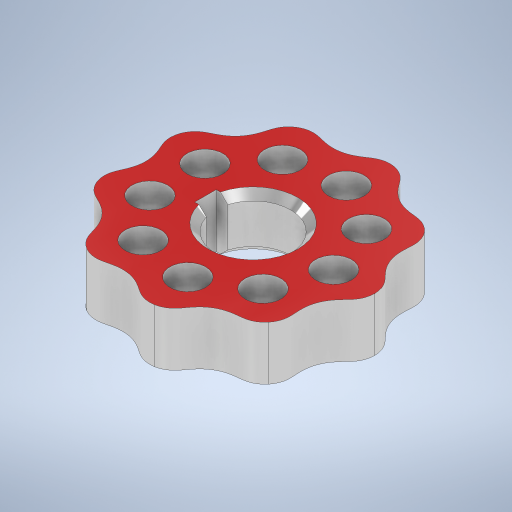
# Autodesk Inventor part: Przekładnia cykloidalna mimośrodowa
Saved by Autodesk Inventor 2023 (Build 270158000, 158)
## iProperties
Created: 2023-04-01
Part Number: Przekładnia cykloidalna mimośrodowa
Material: Stal
Document SubType Name: Modeling
Designer: Wiktor
Density: 7.85 g/cm^3
Appearance: Chrom — polerowany
Author: Wiktor
Autodesk Inventor part; units mm, degrees
ref_plane "YZ Plane" through (0, 0, 0) normal (1, 0, 0) x (0, 1, 0)
ref_plane "XZ Plane" through (0, 0, 0) normal (0, 1, 0) x (-1, 0, 0)
ref_plane "XY Plane" through (0, 0, 0) normal (0, 0, 1) x (1, 0, 0)
sketch "Szkic1" plane through (0, 0, 0) normal (0, 1, 0) x (-1, 0, 0)
  circle A0 centre (0, 0) radius 50
  dimension "d0" = 100
  constraints: 1 centre point, 1 coincident
  measures "d0" diameter of A0
extrude "Wyciągnięcie proste1" add sketch "Szkic1" along normal blind 15
sketch "Szkic2" plane through (0, 15, 0) normal (0, 1, 0) x (1, 0, 0)
  circle A0 centre (0, 0) radius 36 construction
  circle A1 centre (40, 0) radius 4 construction
  circle A2 centre (0, 0) radius 42 construction
  spline S0 degree 5 poles (42, 0) (42.0015, 1.5779) (41.7865, 3.1702) (41.3842, 4.6891) (40.322, 7.2003) (38.7977, 9.322) (38.0479, 10.2329) (36.9029, 11.2622) (35.7039, 12.7118) (35.5218, 13.2122) (35.5085, 15.0934) (35.724, 16.6179) (35.7128, 17.7976) (35.5167, 20.4027) (34.7162, 23.0092) (34.048, 24.4313) (33.1892, 25.7893) (32.1739, 26.9971) knots 0 0 0 0 0 0 0.266019 0.266019 0.266019 0.44748 0.44748 0.44748 0.55252 0.55252 0.55252 0.733981 0.733981 0.733981 1 1 1 1 1 1
  dimension "d3" = 72
  dimension "d4" = 8
  dimension "d5" = 2
  dimension "d6" = 84
  dimension "d11" = 360
  constraints: 3 centre point, 2 coincident, 2 horizontal alignment, 2 point on circle, 1 tangent, 1 vertical alignment, 36 other
  measures "d3" diameter of A0
  measures "d4" diameter of A1
  measures "d5" distance of A1.centre A2.start
  measures "d6" diameter of A2
sketch "Szkic3" plane through (0, 0, 0) normal (0, -1, 0) x (1, 0, 0)
  spline S0 degree 3 poles (7.2932, -41.3619) (5.0487, -41.7577) (2.7266, -41.598) (0.7774, -41.0654) (-1.1614, -40.5357) (-2.7091, -39.6698) (-3.8378, -38.9372) (-5.0099, -38.1765) (-5.75, -37.5995) (-6.519, -37.4381) (-7.2644, -37.2816) (-8.0785, -37.5077) (-9.3169, -37.8082) (-10.5416, -38.1053) (-12.1918, -38.4379) (-14.1354, -38.3619) (-16.0802, -38.2858) (-18.2905, -37.7748) (-20.3, -36.7528) (-20.5364, -36.6326) (-20.77, -36.5059) (-21, -36.3731) knots 0 0 0 0 0.113958 0.113958 0.113958 0.227304 0.227304 0.227304 0.345011 0.345011 0.345011 0.459109 0.459109 0.459109 0.571947 0.571947 0.571947 0.68485 0.68485 0.68485 0.698132 0.698132 0.698132 0.698132 projected
  spline S1 degree 3 poles (32.1739, -26.9971) (30.7089, -28.743) (28.8273, -30.1133) (26.9918, -30.9582) (25.1662, -31.7987) (23.4239, -32.1302) (22.0884, -32.2945) (20.7016, -32.4652) (19.7638, -32.4989) (19.0709, -32.8695) (18.3993, -33.2288) (17.9209, -33.9253) (17.1655, -34.9515) (16.4183, -35.9664) (15.368, -37.2819) (13.8302, -38.473) (12.2915, -39.6648) (10.2699, -40.6941) (8.0736, -41.2029) (7.8152, -41.2627) (7.5548, -41.3158) (7.2932, -41.3619) knots 0 0 0 0 0.113958 0.113958 0.113958 0.227304 0.227304 0.227304 0.345011 0.345011 0.345011 0.459109 0.459109 0.459109 0.571947 0.571947 0.571947 0.68485 0.68485 0.68485 0.698132 0.698132 0.698132 0.698132 projected
  spline S2 degree 3 poles (42, 0) (42, -2.2792) (41.4395, -4.5382) (40.5765, -6.3654) (39.7182, -8.1827) (38.5967, -9.5565) (37.6792, -10.5409) (36.7265, -11.563) (36.0298, -12.1917) (35.7373, -12.921) (35.4538, -13.6279) (35.535, -14.4689) (35.6159, -15.7407) (35.6959, -16.9984) (35.7369, -18.6812) (35.3245, -20.5821) (34.9119, -22.4842) (34.0248, -24.5721) (32.6694, -26.3736) (32.51, -26.5856) (32.3446, -26.7936) (32.1739, -26.9971) knots 0 0 0 0 0.113958 0.113958 0.113958 0.227304 0.227304 0.227304 0.345011 0.345011 0.345011 0.459109 0.459109 0.459109 0.571947 0.571947 0.571947 0.68485 0.68485 0.68485 0.698132 0.698132 0.698132 0.698132 projected
  spline S3 degree 3 poles (32.1739, 26.9971) (33.6389, 25.2511) (34.6616, 23.1603) (35.175, 21.2059) (35.6856, 19.2621) (35.7096, 17.4887) (35.6395, 16.145) (35.5667, 14.7495) (35.4371, 13.8201) (35.6818, 13.0734) (35.919, 12.3496) (36.5219, 11.7576) (37.4013, 10.8354) (38.271, 9.9234) (39.3841, 8.6606) (40.2901, 6.9393) (41.1966, 5.2171) (41.8592, 3.0474) (41.9789, 0.7961) (41.9929, 0.5313) (42, 0.2656) (42, 0) knots 0 0 0 0 0.113958 0.113958 0.113958 0.227304 0.227304 0.227304 0.345011 0.345011 0.345011 0.459109 0.459109 0.459109 0.571947 0.571947 0.571947 0.68485 0.68485 0.68485 0.698132 0.698132 0.698132 0.698132 projected
  spline S4 degree 3 poles (7.2932, 41.3619) (9.5378, 40.9662) (11.6652, 40.0218) (13.3147, 38.8547) (14.9554, 37.6939) (16.1136, 36.3508) (16.9237, 35.2764) (17.7649, 34.1607) (18.263, 33.3654) (18.9304, 32.9507) (19.5774, 32.5487) (20.4197, 32.4826) (21.6862, 32.3415) (22.9386, 32.2019) (24.6031, 31.95) (26.4035, 31.2138) (28.205, 30.4771) (30.1072, 29.241) (31.6459, 27.5933) (31.827, 27.3995) (32.0031, 27.2006) (32.1739, 26.9971) knots 0 0 0 0 0.113958 0.113958 0.113958 0.227304 0.227304 0.227304 0.345011 0.345011 0.345011 0.459109 0.459109 0.459109 0.571947 0.571947 0.571947 0.68485 0.68485 0.68485 0.698132 0.698132 0.698132 0.698132 projected
  spline S5 degree 3 poles (-21, 36.3731) (-19.0262, 37.5126) (-16.7895, 38.1567) (-14.7757, 38.323) (-12.7727, 38.4883) (-11.0221, 38.204) (-9.711, 37.9016) (-8.3494, 37.5876) (-7.4566, 37.2986) (-6.6787, 37.4099) (-5.9248, 37.5178) (-5.237, 38.0087) (-4.1761, 38.7146) (-3.1269, 39.4127) (-1.69, 40.2897) (0.1624, 40.883) (2.0159, 41.4766) (4.2677, 41.7524) (6.5055, 41.4793) (6.7688, 41.4472) (7.0316, 41.4081) (7.2932, 41.3619) knots 0 0 0 0 0.113958 0.113958 0.113958 0.227304 0.227304 0.227304 0.345011 0.345011 0.345011 0.459109 0.459109 0.459109 0.571947 0.571947 0.571947 0.68485 0.68485 0.68485 0.698132 0.698132 0.698132 0.698132 projected
  spline S6 degree 3 poles (-39.4671, 14.3648) (-38.6876, 16.5065) (-37.3882, 18.4377) (-35.9524, 19.8595) (-34.5242, 21.2736) (-33.0005, 22.181) (-31.8017, 22.7922) (-30.5568, 23.4269) (-29.6871, 23.7794) (-29.1628, 24.3646) (-28.6546, 24.9319) (-28.4433, 25.7501) (-28.0844, 26.9728) (-27.7294, 28.182) (-27.1923, 29.7773) (-26.1547, 31.4226) (-25.1164, 33.0688) (-23.5687, 34.7274) (-21.6789, 35.9567) (-21.4566, 36.1013) (-21.23, 36.2402) (-21, 36.3731) knots 0 0 0 0 0.113958 0.113958 0.113958 0.227304 0.227304 0.227304 0.345011 0.345011 0.345011 0.459109 0.459109 0.459109 0.571947 0.571947 0.571947 0.68485 0.68485 0.68485 0.698132 0.698132 0.698132 0.698132 projected
  spline S7 degree 3 poles (-39.4671, -14.3648) (-40.2466, -12.2231) (-40.4925, -9.9086) (-40.3065, -7.8965) (-40.1215, -5.8952) (-39.5375, -4.2206) (-39.0121, -2.9819) (-38.4664, -1.6955) (-38.0268, -0.8665) (-38.0013, -0.0811) (-37.9766, 0.6801) (-38.3407, 1.4427) (-38.8516, 2.61) (-39.357, 3.7645) (-39.971, 5.3319) (-40.2337, 7.2592) (-40.4965, 9.1876) (-40.377, 11.4531) (-39.7195, 13.6095) (-39.6422, 13.8632) (-39.5579, 14.1152) (-39.4671, 14.3648) knots 0 0 0 0 0.113958 0.113958 0.113958 0.227304 0.227304 0.227304 0.345011 0.345011 0.345011 0.459109 0.459109 0.459109 0.571947 0.571947 0.571947 0.68485 0.68485 0.68485 0.698132 0.698132 0.698132 0.698132 projected
  spline S8 degree 3 poles (-21, -36.3731) (-22.9738, -35.2335) (-24.65, -33.6185) (-25.8008, -31.9576) (-26.9455, -30.3056) (-27.5745, -28.6474) (-27.9683, -27.3607) (-28.3771, -26.0246) (-28.5732, -25.1069) (-29.0586, -24.4889) (-29.529, -23.8899) (-30.298, -23.5397) (-31.4398, -22.9739) (-32.569, -22.4144) (-34.0469, -21.6084) (-35.4869, -20.3008) (-36.9278, -18.9925) (-38.2925, -17.1803) (-39.1749, -15.1057) (-39.2787, -14.8617) (-39.3762, -14.6145) (-39.4671, -14.3648) knots 0 0 0 0 0.113958 0.113958 0.113958 0.227304 0.227304 0.227304 0.345011 0.345011 0.345011 0.459109 0.459109 0.459109 0.571947 0.571947 0.571947 0.68485 0.68485 0.68485 0.698132 0.698132 0.698132 0.698132 projected
  circle A0 centre (0, 0) radius 50 projected
extrude "Wyciągnięcie proste2" cut sketch "Szkic3" against normal blind 15
sketch "Szkic4" plane through (0, 0, 0) normal (0, -1, 0) x (1, 0, 0)
  spline S0 degree 3 poles (-21, -36.3731) (-22.9738, -35.2335) (-24.65, -33.6185) (-25.8008, -31.9576) (-26.9455, -30.3056) (-27.5745, -28.6474) (-27.9683, -27.3607) (-28.3771, -26.0246) (-28.5732, -25.1069) (-29.0586, -24.4889) (-29.529, -23.8899) (-30.298, -23.5397) (-31.4398, -22.9739) (-32.569, -22.4144) (-34.0469, -21.6084) (-35.4869, -20.3008) (-36.9278, -18.9925) (-38.2925, -17.1803) (-39.1749, -15.1057) (-39.2787, -14.8617) (-39.3762, -14.6145) (-39.4671, -14.3648) knots 0 0 0 0 0.163232 0.163232 0.163232 0.325589 0.325589 0.325589 0.494192 0.494192 0.494192 0.657625 0.657625 0.657625 0.819254 0.819254 0.819254 0.980975 0.980975 0.980975 1 1 1 1 projected
  spline S1 degree 3 poles (-39.4671, -14.3648) (-40.2466, -12.2231) (-40.4925, -9.9086) (-40.3065, -7.8965) (-40.1215, -5.8952) (-39.5375, -4.2206) (-39.0121, -2.9819) (-38.4664, -1.6955) (-38.0268, -0.8665) (-38.0013, -0.0811) (-37.9766, 0.6801) (-38.3407, 1.4427) (-38.8516, 2.61) (-39.357, 3.7645) (-39.971, 5.3319) (-40.2337, 7.2592) (-40.4965, 9.1876) (-40.377, 11.4531) (-39.7195, 13.6095) (-39.6422, 13.8632) (-39.5579, 14.1152) (-39.4671, 14.3648) knots 0 0 0 0 0.163232 0.163232 0.163232 0.325589 0.325589 0.325589 0.494192 0.494192 0.494192 0.657625 0.657625 0.657625 0.819254 0.819254 0.819254 0.980975 0.980975 0.980975 1 1 1 1 projected
  spline S2 degree 3 poles (-39.4671, 14.3648) (-38.6876, 16.5065) (-37.3882, 18.4377) (-35.9524, 19.8595) (-34.5242, 21.2736) (-33.0005, 22.181) (-31.8017, 22.7922) (-30.5568, 23.4269) (-29.6871, 23.7794) (-29.1628, 24.3646) (-28.6546, 24.9319) (-28.4433, 25.7501) (-28.0844, 26.9728) (-27.7294, 28.182) (-27.1923, 29.7773) (-26.1547, 31.4226) (-25.1164, 33.0688) (-23.5687, 34.7274) (-21.6789, 35.9567) (-21.4566, 36.1013) (-21.23, 36.2402) (-21, 36.3731) knots 0 0 0 0 0.163232 0.163232 0.163232 0.325589 0.325589 0.325589 0.494192 0.494192 0.494192 0.657625 0.657625 0.657625 0.819254 0.819254 0.819254 0.980975 0.980975 0.980975 1 1 1 1 projected
  spline S3 degree 3 poles (-21, 36.3731) (-19.0262, 37.5126) (-16.7895, 38.1567) (-14.7757, 38.323) (-12.7727, 38.4883) (-11.0221, 38.204) (-9.711, 37.9016) (-8.3494, 37.5876) (-7.4566, 37.2986) (-6.6787, 37.4099) (-5.9248, 37.5178) (-5.237, 38.0087) (-4.1761, 38.7146) (-3.1269, 39.4127) (-1.69, 40.2897) (0.1624, 40.883) (2.0159, 41.4766) (4.2677, 41.7524) (6.5055, 41.4793) (6.7688, 41.4472) (7.0316, 41.4081) (7.2932, 41.3619) knots 0 0 0 0 0.163232 0.163232 0.163232 0.325589 0.325589 0.325589 0.494192 0.494192 0.494192 0.657625 0.657625 0.657625 0.819254 0.819254 0.819254 0.980975 0.980975 0.980975 1 1 1 1 projected
  spline S4 degree 3 poles (7.2932, 41.3619) (9.5378, 40.9662) (11.6652, 40.0218) (13.3147, 38.8547) (14.9554, 37.6939) (16.1136, 36.3508) (16.9237, 35.2764) (17.7649, 34.1607) (18.263, 33.3654) (18.9304, 32.9507) (19.5774, 32.5487) (20.4197, 32.4826) (21.6862, 32.3415) (22.9386, 32.2019) (24.6031, 31.95) (26.4035, 31.2138) (28.205, 30.4771) (30.1072, 29.241) (31.6459, 27.5933) (31.827, 27.3995) (32.0031, 27.2006) (32.1739, 26.9971) knots 0 0 0 0 0.163232 0.163232 0.163232 0.325589 0.325589 0.325589 0.494192 0.494192 0.494192 0.657625 0.657625 0.657625 0.819254 0.819254 0.819254 0.980975 0.980975 0.980975 1 1 1 1 projected
  spline S5 degree 3 poles (32.1739, 26.9971) (33.6389, 25.2511) (34.6616, 23.1603) (35.175, 21.2059) (35.6856, 19.2621) (35.7096, 17.4887) (35.6395, 16.145) (35.5667, 14.7495) (35.4371, 13.8201) (35.6818, 13.0734) (35.919, 12.3496) (36.5219, 11.7576) (37.4013, 10.8354) (38.271, 9.9234) (39.3841, 8.6606) (40.2901, 6.9393) (41.1966, 5.2171) (41.8592, 3.0474) (41.9789, 0.7961) (41.9929, 0.5313) (42, 0.2656) (42, 0) knots 0 0 0 0 0.163232 0.163232 0.163232 0.325589 0.325589 0.325589 0.494192 0.494192 0.494192 0.657625 0.657625 0.657625 0.819254 0.819254 0.819254 0.980975 0.980975 0.980975 1 1 1 1 projected
  spline S6 degree 3 poles (42, 0) (42, -2.2792) (41.4395, -4.5382) (40.5765, -6.3654) (39.7182, -8.1827) (38.5967, -9.5565) (37.6792, -10.5409) (36.7265, -11.563) (36.0298, -12.1917) (35.7373, -12.921) (35.4538, -13.6279) (35.535, -14.4689) (35.6159, -15.7407) (35.6959, -16.9984) (35.7369, -18.6812) (35.3245, -20.5821) (34.9119, -22.4842) (34.0248, -24.5721) (32.6694, -26.3736) (32.51, -26.5856) (32.3446, -26.7936) (32.1739, -26.9971) knots 0 0 0 0 0.163232 0.163232 0.163232 0.325589 0.325589 0.325589 0.494192 0.494192 0.494192 0.657625 0.657625 0.657625 0.819254 0.819254 0.819254 0.980975 0.980975 0.980975 1 1 1 1 projected
  spline S7 degree 3 poles (32.1739, -26.9971) (30.7089, -28.743) (28.8273, -30.1133) (26.9918, -30.9582) (25.1662, -31.7987) (23.4239, -32.1302) (22.0884, -32.2945) (20.7016, -32.4652) (19.7638, -32.4989) (19.0709, -32.8695) (18.3993, -33.2288) (17.9209, -33.9253) (17.1655, -34.9515) (16.4183, -35.9664) (15.368, -37.2819) (13.8302, -38.473) (12.2915, -39.6648) (10.2699, -40.6941) (8.0736, -41.2029) (7.8152, -41.2627) (7.5548, -41.3158) (7.2932, -41.3619) knots 0 0 0 0 0.163232 0.163232 0.163232 0.325589 0.325589 0.325589 0.494192 0.494192 0.494192 0.657625 0.657625 0.657625 0.819254 0.819254 0.819254 0.980975 0.980975 0.980975 1 1 1 1 projected
  spline S8 degree 3 poles (7.2932, -41.3619) (5.0487, -41.7577) (2.7266, -41.598) (0.7774, -41.0654) (-1.1614, -40.5357) (-2.7091, -39.6698) (-3.8378, -38.9372) (-5.0099, -38.1765) (-5.75, -37.5995) (-6.519, -37.4381) (-7.2644, -37.2816) (-8.0785, -37.5077) (-9.3169, -37.8082) (-10.5416, -38.1053) (-12.1918, -38.4379) (-14.1354, -38.3619) (-16.0802, -38.2858) (-18.2905, -37.7748) (-20.3, -36.7528) (-20.5364, -36.6326) (-20.77, -36.5059) (-21, -36.3731) knots 0 0 0 0 0.163232 0.163232 0.163232 0.325589 0.325589 0.325589 0.494192 0.494192 0.494192 0.657625 0.657625 0.657625 0.819254 0.819254 0.819254 0.980975 0.980975 0.980975 1 1 1 1 projected
  spline S9 degree 5 poles (5.904, 33.4835) (5.5616, 33.5437) (5.2153, 33.5847) (4.8666, 33.596) (4.1943, 33.5839) (3.5277, 33.4945) (3.2089, 33.436) (2.6122, 33.2885) (2.0406, 33.0643) (1.7757, 32.9466) (1.2221, 32.6654) (0.6904, 32.3441) (0.4138, 32.1618) (-0.3628, 31.6382) (-1.1466, 31.1255) (-1.6678, 30.8155) (-3.1223, 30.0628) (-4.6904, 29.5698) (-5.7165, 29.3876) (-7.3568, 29.3161) (-8.9781, 29.5284) (-9.5717, 29.6411) (-10.4783, 29.8572) (-11.3838, 30.0788) (-11.7035, 30.1572) (-12.3159, 30.2772) (-12.9352, 30.3506) (-13.2293, 30.3714) (-13.8419, 30.3848) (-14.4523, 30.3262) (-14.766, 30.2707) (-15.4195, 30.1253) (-16.053, 29.9064) (-16.3787, 29.7738) (-16.6958, 29.6203) (-17, 29.4449) knots 0 0 0 0 0 0 0.072134 0.072134 0.072134 0.13926 0.13926 0.13926 0.199279 0.199279 0.199279 0.267978 0.267978 0.267978 0.393538 0.393538 0.393538 0.606919 0.606919 0.606919 0.73199 0.73199 0.73199 0.800252 0.800252 0.800252 0.861284 0.861284 0.861284 0.927161 0.927161 0.927161 1 1 1 1 1 1
  spline S10 degree 5 poles (-17, 29.4449) (-17.3011, 29.2709) (-17.5927, 29.0797) (-17.8671, 28.8643) (-18.3743, 28.4228) (-18.8275, 27.9258) (-19.034, 27.6761) (-19.3964, 27.1796) (-19.6902, 26.6404) (-19.8174, 26.3799) (-20.0607, 25.8086) (-20.2615, 25.2208) (-20.3562, 24.9033) (-20.6146, 24.003) (-20.8855, 23.1065) (-21.0854, 22.534) (-21.7158, 21.0224) (-22.6001, 19.6368) (-23.2691, 18.8377) (-24.4797, 17.7285) (-25.8581, 16.8491) (-26.3853, 16.5539) (-27.2187, 16.1366) (-28.0548, 15.7243) (-28.3501, 15.5789) (-28.8964, 15.2772) (-29.418, 14.9353) (-29.6567, 14.7622) (-30.1345, 14.3788) (-30.5644, 13.9414) (-30.769, 13.6973) (-31.1762, 13.1658) (-31.5207, 12.5909) (-31.6851, 12.2801) (-31.8293, 11.9586) (-31.9495, 11.6287) knots 0 0 0 0 0 0 0.072134 0.072134 0.072134 0.13926 0.13926 0.13926 0.199279 0.199279 0.199279 0.267978 0.267978 0.267978 0.393538 0.393538 0.393538 0.606919 0.606919 0.606919 0.73199 0.73199 0.73199 0.800252 0.800252 0.800252 0.861284 0.861284 0.861284 0.927161 0.927161 0.927161 1 1 1 1 1 1
  spline S11 degree 5 poles (-31.9495, 11.6287) (-32.0683, 11.3019) (-32.1689, 10.968) (-32.2406, 10.6266) (-32.3454, 9.9623) (-32.3731, 9.2903) (-32.3708, 8.9663) (-32.3292, 8.353) (-32.2076, 7.7511) (-32.1377, 7.4698) (-31.9569, 6.8758) (-31.7329, 6.2964) (-31.6013, 5.9923) (-31.2205, 5.1366) (-30.8518, 4.2757) (-30.6369, 3.7086) (-30.1482, 2.1455) (-29.935, 0.5156) (-29.9338, -0.5266) (-30.1482, -2.1544) (-30.6389, -3.7141) (-30.8529, -4.2791) (-31.2231, -5.1345) (-31.5986, -5.9877) (-31.7313, -6.289) (-31.9559, -6.8712) (-32.1357, -7.4684) (-32.2073, -7.7544) (-32.3268, -8.3553) (-32.3751, -8.9667) (-32.3749, -9.2852) (-32.3452, -9.9541) (-32.2396, -10.6159) (-32.1656, -10.9597) (-32.0695, -11.2987) (-31.9495, -11.6287) knots 0 0 0 0 0 0 0.072134 0.072134 0.072134 0.13926 0.13926 0.13926 0.199279 0.199279 0.199279 0.267978 0.267978 0.267978 0.393538 0.393538 0.393538 0.606919 0.606919 0.606919 0.73199 0.73199 0.73199 0.800252 0.800252 0.800252 0.861284 0.861284 0.861284 0.927161 0.927161 0.927161 1 1 1 1 1 1
  spline S12 degree 5 poles (-31.9495, -11.6287) (-31.8305, -11.9554) (-31.6929, -12.2758) (-31.5283, -12.5834) (-31.1817, -13.1596) (-30.7709, -13.6922) (-30.5608, -13.939) (-30.1348, -14.382) (-29.6548, -14.765) (-29.4204, -14.9355) (-28.9001, -15.2743) (-28.356, -15.5742) (-28.0598, -15.7225) (-27.2181, -16.1333) (-26.3822, -16.5558) (-25.8531, -16.8521) (-24.474, -17.7354) (-23.263, -18.8469) (-22.5922, -19.6444) (-21.7101, -21.0292) (-21.0833, -22.5395) (-20.8841, -23.1099) (-20.6179, -24.0031) (-20.3571, -24.8981) (-20.2652, -25.2141) (-20.0629, -25.8045) (-19.8168, -26.3776) (-19.6878, -26.6427) (-19.3931, -27.1798) (-19.0371, -27.6792) (-18.8322, -27.9231) (-18.3795, -28.4163) (-17.8732, -28.8555) (-17.5955, -29.0713) (-17.304, -29.2692) (-17, -29.4449) knots 0 0 0 0 0 0 0.072134 0.072134 0.072134 0.13926 0.13926 0.13926 0.199279 0.199279 0.199279 0.267978 0.267978 0.267978 0.393538 0.393538 0.393538 0.606919 0.606919 0.606919 0.73199 0.73199 0.73199 0.800252 0.800252 0.800252 0.861284 0.861284 0.861284 0.927161 0.927161 0.927161 1 1 1 1 1 1
  spline S13 degree 5 poles (-17, -29.4449) (-16.6988, -29.6186) (-16.3874, -29.7756) (-16.0637, -29.9055) (-15.4277, -30.124) (-14.7707, -30.268) (-14.4512, -30.322) (-13.84, -30.3875) (-13.2261, -30.3724) (-12.937, -30.3524) (-12.3206, -30.2774) (-11.7111, -30.1574) (-11.3888, -30.0807) (-10.48, -29.8542) (-9.5681, -29.6406) (-8.9723, -29.5275) (-7.3481, -29.3176) (-5.7059, -29.3907) (-4.6794, -29.5705) (-3.1135, -30.0643) (-1.6627, -30.8184) (-1.1434, -31.1273) (-0.3653, -31.6404) (0.4097, -32.1583) (0.6833, -32.3413) (1.2178, -32.6636) (1.7746, -32.9444) (2.0439, -33.0645) (2.6149, -33.2866) (3.2086, -33.4403) (3.5223, -33.4954) (4.1861, -33.5823) (4.8563, -33.5932) (5.2077, -33.5801) (5.5582, -33.5443) (5.904, -33.4835) knots 0 0 0 0 0 0 0.072134 0.072134 0.072134 0.13926 0.13926 0.13926 0.199279 0.199279 0.199279 0.267978 0.267978 0.267978 0.393538 0.393538 0.393538 0.606919 0.606919 0.606919 0.73199 0.73199 0.73199 0.800252 0.800252 0.800252 0.861284 0.861284 0.861284 0.927161 0.927161 0.927161 1 1 1 1 1 1
  spline S14 degree 5 poles (5.904, -33.4835) (6.2464, -33.4229) (6.5859, -33.3431) (6.9174, -33.2344) (7.545, -32.9931) (8.1409, -32.6811) (8.4204, -32.517) (8.9307, -32.1744) (9.3912, -31.7682) (9.5998, -31.567) (10.0239, -31.1134) (10.4136, -30.6297) (10.6111, -30.3637) (11.1618, -29.6061) (11.7231, -28.8563) (12.1067, -28.3866) (13.2161, -27.1819) (14.521, -26.1823) (15.4229, -25.6602) (16.9398, -25.0319) (18.536, -24.677) (19.1323, -24.5798) (20.0582, -24.4727) (20.9848, -24.3714) (21.3121, -24.3357) (21.9286, -24.239) (22.5357, -24.0962) (22.8192, -24.0151) (23.3993, -23.8182) (23.9529, -23.5543) (24.2287, -23.3949) (24.7931, -23.0347) (25.3135, -22.6123) (25.5742, -22.3764) (25.8197, -22.1237) (26.0455, -21.8548) knots 0 0 0 0 0 0 0.072134 0.072134 0.072134 0.13926 0.13926 0.13926 0.199279 0.199279 0.199279 0.267978 0.267978 0.267978 0.393538 0.393538 0.393538 0.606919 0.606919 0.606919 0.73199 0.73199 0.73199 0.800252 0.800252 0.800252 0.861284 0.861284 0.861284 0.927161 0.927161 0.927161 1 1 1 1 1 1
  spline S15 degree 5 poles (26.0455, -21.8548) (26.2689, -21.5883) (26.4776, -21.3089) (26.6617, -21.0126) (26.9874, -20.4243) (27.2433, -19.8023) (27.3519, -19.497) (27.5226, -18.9065) (27.6142, -18.2993) (27.6448, -18.0111) (27.678, -17.391) (27.6657, -16.77) (27.646, -16.4392) (27.5809, -15.5049) (27.5288, -14.5697) (27.5209, -13.9634) (27.5963, -12.3274) (27.9533, -10.7229) (28.3087, -9.7432) (29.0669, -8.2869) (30.0614, -6.989) (30.4558, -6.5312) (31.0962, -5.8541) (31.7409, -5.1808) (31.9686, -4.9431) (32.3788, -4.4727) (32.752, -3.9731) (32.9171, -3.7288) (33.235, -3.205) (33.4894, -2.647) (33.5982, -2.3476) (33.799, -1.709) (33.9262, -1.0509) (33.9743, -0.7025) (33.9999, -0.3511) (34, 0) knots 0 0 0 0 0 0 0.072134 0.072134 0.072134 0.13926 0.13926 0.13926 0.199279 0.199279 0.199279 0.267978 0.267978 0.267978 0.393538 0.393538 0.393538 0.606919 0.606919 0.606919 0.73199 0.73199 0.73199 0.800252 0.800252 0.800252 0.861284 0.861284 0.861284 0.927161 0.927161 0.927161 1 1 1 1 1 1
  spline S16 degree 5 poles (34, 0) (33.9998, 0.3477) (33.9801, 0.6959) (33.9307, 1.0412) (33.802, 1.7012) (33.5982, 2.3422) (33.4852, 2.6459) (33.2364, 3.208) (32.9163, 3.732) (32.7544, 3.9724) (32.3813, 4.4688) (31.9727, 4.9366) (31.745, 5.1773) (31.0945, 5.8512) (30.4535, 6.5341) (30.0577, 6.9935) (29.0639, 8.2952) (28.306, 9.7539) (27.9485, 10.7328) (27.5932, 12.3357) (27.5208, 13.9693) (27.5287, 14.5734) (27.584, 15.5038) (27.6451, 16.434) (27.6668, 16.7624) (27.6786, 17.3864) (27.6434, 18.0091) (27.6128, 18.3023) (27.5196, 18.9079) (27.3558, 19.4989) (27.2467, 19.7981) (26.9901, 20.4165) (26.6644, 21.0023) (26.4774, 21.3001) (26.2711, 21.5857) (26.0455, 21.8548) knots 0 0 0 0 0 0 0.072134 0.072134 0.072134 0.13926 0.13926 0.13926 0.199279 0.199279 0.199279 0.267978 0.267978 0.267978 0.393538 0.393538 0.393538 0.606919 0.606919 0.606919 0.73199 0.73199 0.73199 0.800252 0.800252 0.800252 0.861284 0.861284 0.861284 0.927161 0.927161 0.927161 1 1 1 1 1 1
  spline S17 degree 5 poles (26.0455, 21.8548) (25.8219, 22.121) (25.583, 22.3751) (25.3232, 22.6079) (24.8003, 23.0307) (24.2322, 23.3907) (23.9504, 23.5508) (23.3985, 23.8214) (22.8165, 24.0171) (22.5379, 24.0972) (21.933, 24.2376) (21.3193, 24.3333) (20.9902, 24.3714) (20.0587, 24.4695) (19.1287, 24.5806) (18.5302, 24.6781) (16.9322, 25.0364) (15.414, 25.6667) (14.5109, 26.1867) (13.2084, 27.1863) (12.1029, 28.3911) (11.7206, 28.859) (11.1649, 29.6073) (10.6138, 30.3591) (10.4193, 30.6246) (10.0273, 31.1102) (9.6, 31.5645) (9.3881, 31.7695) (8.9275, 32.1735) (8.4222, 32.521) (8.1462, 32.6801) (7.5521, 32.9888) (6.9261, 33.2283) (6.5914, 33.3361) (6.2498, 33.4224) (5.904, 33.4835) knots 0 0 0 0 0 0 0.072134 0.072134 0.072134 0.13926 0.13926 0.13926 0.199279 0.199279 0.199279 0.267978 0.267978 0.267978 0.393538 0.393538 0.393538 0.606919 0.606919 0.606919 0.73199 0.73199 0.73199 0.800252 0.800252 0.800252 0.861284 0.861284 0.861284 0.927161 0.927161 0.927161 1 1 1 1 1 1
  point P0 (0, 0)
  dimension "d15" = 8
  constraints: 2 vertical alignment, 34 other
extrude "Wyciągnięcie proste3" cut sketch "Szkic4" against normal blind 15
sketch "Szkic5" plane through (0, 0, 0) normal (0, -1, 0) x (1, 0, 0)
  arc A0 (-10.0623, -3) -> (-10.0623, 3) centre (0, 0) ccw
  circle A1 centre (0, 0) radius 22.5 construction
  circle A2 centre (22.5, 0) radius 5
  line L0 (-10.0623, 3) -> (-13.3, 3)
  line L1 (-13.3, 3) -> (-13.3, -3)
  line L2 (-13.3, -3) -> (-10.0623, -3)
  point P0 (-13.3, 0)
  point P1 (10.5, 0)
  dimension "d19" = 45
  dimension "d18" = 21
  dimension "d20" = 10
  dimension "d21" = 6
  dimension "d22" = 23.8
  dimension "d23" = 0
  constraints: 6 end point, 3 horizontal alignment, 3 point on circle, 2 centre point, 2 coincident, 2 perpendicular, 1 horizontal, 1 midpoint, 2 other
  measures "d18" diameter of A0
  measures "d20" diameter of A2
  measures "d21" distance of L0.end L1.end
  measures "d22" distance from line of point (10.5, 0) L1
  measures "d23" distance of A0.centre point (0, 0)
extrude "Wyciągnięcie proste4" cut sketch "Szkic5" against normal blind 15 contours A2
pattern_circular "Szyk kołowy1" count 9 over 360 about axis through (0, -10, 0) along (0, 1, 0) of "Wyciągnięcie proste4"
extrude "Wyciągnięcie proste5" cut sketch "Szkic5" against normal blind 15 contours L2 L1 L0 A0
chamfer "Faza1" distance 2 angle 45 2 edges at (10.5, 0, 0) (10.5, 15, 0)
sketch "Szkic6" plane through (0, 0, 0) normal (0, -1, 0) x (1, 0, 0)
  point P0 (0, 0)
sketch "Szkic7" plane through (0, 0, 0) normal (0, -1, 0) x (1, 0, 0)
  line L0 (-31.9495, 11.6287) -> (0, 0)
  constraints: 2 end point
equation "curve S0 of \"Szkic2\": x = 40*cos(1rad*t)+2*cos(1rad*40*t/4); y = 40*sin(1rad*t)+2*sin(1rad* 40*t/4); t from d7 to d8"
